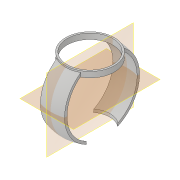
# Autodesk Inventor part: mid_panel
Saved by Autodesk Inventor 2017 (Build 210142000, 142)
## iProperties
Created: 2018-10-19
Part Number: mid_panel
Material: Generic
Document SubType Name: Modeling
Designer: jpb34
Density: 1 g/cm^3
Appearance: Default
Author: jpb34
Autodesk Inventor part; units mm, degrees
ref_plane "XY Plane" through (0, 0, 0) normal (0, 0, 1) x (1, 0, 0)
sketch "Sketch1" plane through (0, 0, 0) normal (0, 1, 0) x (-1, 0, 0)
  circle A0 centre (0, 0) radius 21.59
  line L0 (0, -21.59) -> (0, 21.59)
  dimension "d0" = 43.18
  constraints: 2 end point, 2 point on circle, 1 centre point, 1 coincident, 1 vertical
  measures "d0" diameter of A0
revolve "Revolution1" add sketch "Sketch1" angle 360 about axis through (0, 0, -21.59) along (0, 0, 1)
sketch "Sketch2" plane through (0, 0, 0) normal (0, 1, 0) x (-1, 0, 0)
  line L0 (-6.604, -23.7777) -> (-21.7081, -23.7777)
  line L1 (-21.7081, -23.7777) -> (-21.7081, 23.9273)
  line L2 (-21.7081, 23.9273) -> (-6.604, 23.9273)
  line L3 (-6.604, 23.9273) -> (-6.604, -23.7777)
  line L4 (6.604, 26.32) -> (23.3531, 26.32)
  line L5 (23.3531, 26.32) -> (23.3531, -25.5723)
  line L6 (23.3531, -25.5723) -> (6.604, -25.5723)
  line L7 (6.604, -25.5723) -> (6.604, 26.32)
  point P0 (0, 0)
  dimension "d2" = 6.604
  dimension "d3" = 6.604
  constraints: 16 end point, 4 parallel, 2 horizontal, 2 perpendicular
  measures "d2" distance from line of point (0, 0) L3
  measures "d3" distance from line of L7 point (0, 0)
extrude "Extrusion1" cut sketch "Sketch2" along normal mid plane 50.8
sketch "Sketch3" plane through (0, 0, 0) normal (0, 1, 0) x (-1, 0, 0)
  circle A0 centre (0, 0) radius 12.446
  dimension "d6" = 24.892
  constraints: 1 centre point, 1 coincident
  measures "d6" diameter of A0
extrude "Extrusion2" cut sketch "Sketch3" along normal blind 47.625 and the other way blind 22.2377 draft -5
sketch "Sketch4" plane through (0, 0, 0) normal (0, 1, 0) x (-1, 0, 0)
  circle A0 centre (0, 0) radius 20.32
  line L0 (20.32, 0) -> (-20.32, 0)
  dimension "d11" = 40.64
  constraints: 2 end point, 2 point on circle, 1 centre point, 1 coincident, 1 horizontal
  measures "d11" diameter of A0
revolve "Revolution2" cut sketch "Sketch4" angle 360 about axis through (-20.32, 0, 0) along (1, 0, 0)
sketch "Sketch5" plane through (0, 0, 0) normal (0, 1, 0) x (-1, 0, 0)
  circle A0 centre (0, 0) radius 13.3548
  circle A1 centre (0, 0) radius 12.446
  constraints: 2 centre point, 2 coincident
extrude "Extrusion3" add sketch "Sketch5" along normal blind 17.78
sketch "Sketch6" plane through (0, 0, 0) normal (0, 1, 0) x (-1, 0, 0)
  circle A0 centre (0, 0) radius 12.446
  circle A1 centre (0, 0) radius 12.446 projected
  circle A2 centre (0, 0) radius 13.3548
  constraints: 2 centre point, 2 coincident
extrude "Extrusion4" cut sketch "Sketch6" along normal blind 14.732
body "Solid1"
